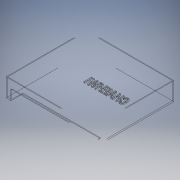
# Autodesk Inventor part: 240621_뚜껑
Saved by Autodesk Inventor 2016 (Build 200138000, 138)
## iProperties
Created: 2024-06-21
Part Number: 240621_뚜껑
Material: 일반
Document SubType Name: Modeling
Designer: pc
Density: 1 g/cm^3
Appearance: 기본값
Author: pc
Autodesk Inventor part; units mm, degrees
ref_plane "YZ Plane" through (0, 0, 0) normal (1, 0, 0) x (0, 1, 0)
ref_plane "XZ Plane" through (0, 0, 0) normal (0, 1, 0) x (-1, 0, 0)
ref_plane "XY Plane" through (0, 0, 0) normal (0, 0, 1) x (1, 0, 0)
sketch "스케치1" plane through (0, 0, 0) normal (0, 0, 1) x (1, 0, 0)
  line L0 (67, -62) -> (-67, -62)
  line L1 (-67, -62) -> (-67, 62)
  line L2 (-67, 62) -> (67, 62)
  line L3 (67, 62) -> (67, -62)
  line L4 (67, -62) -> (-67, 62) construction
  line L5 (-67, -62) -> (67, 62) construction
  point P0 (0, 0)
  dimension "d0" = 134
  dimension "d1" = 124
  constraints: 12 end point, 2 midpoint, 2 parallel, 1 horizontal, 1 perpendicular
  measures "d0" distance of L1.end L2.end
  measures "d1" distance of L0.end L1.end
extrude "돌출1" add sketch "스케치1" along normal blind 28
shell "쉘1" thickness 1.2 removed faces 1 at (22.3333, 20.6667, 28)
sketch "스케치2" plane through (0, 0, 0) normal (0, 0, -1) x (-1, 0, 0)
  line L0 (59.4523, -61.8902) -> (-59.4523, -61.8902)
  line L1 (-59.4523, -61.8902) -> (-59.4523, -43.79)
  line L2 (-59.4523, -43.79) -> (59.4523, -43.79)
  line L3 (59.4523, -43.79) -> (59.4523, -61.8902)
  line L4 (59.4523, -61.8902) -> (-59.4523, -43.79) construction
  line L5 (-59.4523, -61.8902) -> (59.4523, -43.79) construction
  point P0 (0, 0)
  point P1 (0, -52.8401)
  constraints: 12 end point, 2 midpoint, 2 parallel, 1 horizontal, 1 perpendicular
extrude "돌출2" cut sketch "스케치2" against normal blind 1.2
sketch "스케치3" plane through (0, 0, 0) normal (0, 0, -1) x (-1, 0, 0)
  line L0 (-31.3452, 31.9819) -> (-10.2317, 31.9819) construction
  line L1 (-10.2317, 31.9819) -> (-10.2317, 28.3571) construction
  line L2 (-10.2317, 28.3571) -> (-31.3452, 28.3571) construction
  line L3 (-31.3452, 28.3571) -> (-31.3452, 31.9819) construction
  spline S0 degree 2 poles (-23.1755, 23.6344) (-23.1755, 23.7476) (-23.1755, 23.9819) (-23.2078, 24.1597) knots 0 0 0 1 2 2 2
  line L4 (-23.2078, 24.1597) -> (-24.7432, 24.1597)
  spline S1 degree 2 poles (-24.7432, 24.1597) (-24.7432, 23.1981) (-25.325, 20.7657) (-26.7714, 20.7657) knots 0 0 0 1 2 2 2
  spline S2 degree 2 poles (-26.7714, 20.7657) (-28.3068, 20.8789) (-28.9129, 23.8122) (-28.9129, 25.4284) knots 0 0 0 1 2 2 2
  spline S3 degree 2 poles (-28.9129, 25.4284) (-28.9129, 25.5496) (-28.9129, 25.7758) (-28.9129, 25.8971) knots 0 0 0 1 2 2 2
  spline S4 degree 2 poles (-28.9129, 25.8971) (-28.9129, 27.0849) (-28.3472, 30.5597) (-26.828, 30.5597) knots 0 0 0 1 2 2 2
  spline S5 degree 2 poles (-26.828, 30.5597) (-25.4219, 30.5597) (-24.7432, 28.79) (-24.7432, 27.8364) knots 0 0 0 1 2 2 2
  line L5 (-24.7432, 27.8364) -> (-23.2078, 27.8364)
  spline S6 degree 2 poles (-23.2078, 27.8364) (-23.1755, 27.9819) (-23.1755, 28.1516) (-23.1755, 28.2162) knots 0 0 0 1 2 2 2
  spline S7 degree 2 poles (-23.1755, 28.2162) (-23.1755, 30.4142) (-25.325, 31.9819) (-26.6098, 31.9819) knots 0 0 0 1 2 2 2
  spline S8 degree 2 poles (-26.6098, 31.9819) (-29.4785, 31.893) (-30.4805, 27.4001) (-30.4805, 25.4284) knots 0 0 0 1 2 2 2
  spline S9 degree 2 poles (-30.4805, 25.4284) (-30.4805, 22.8829) (-29.131, 19.4567) (-26.6098, 19.3435) knots 0 0 0 1 2 2 2
  spline S10 degree 2 poles (-26.6098, 19.3435) (-24.7512, 19.3435) (-23.1755, 21.9536) (-23.1755, 23.6344) knots 0 0 0 1 2 2 2
  line L6 (-14.0765, 19.6021) -> (-14.0765, 31.6021)
  line L7 (-14.0765, 31.6021) -> (-15.6442, 31.6021)
  line L8 (-15.6442, 31.6021) -> (-15.6442, 26.7617)
  line L9 (-15.6442, 26.7617) -> (-19.927, 26.7617)
  line L10 (-19.927, 26.7617) -> (-19.927, 31.6021)
  line L11 (-19.927, 31.6021) -> (-21.4947, 31.6021)
  line L12 (-21.4947, 31.6021) -> (-21.4947, 19.6021)
  line L13 (-21.4947, 19.6021) -> (-19.927, 19.6021)
  line L14 (-19.927, 19.6021) -> (-19.927, 25.3395)
  line L15 (-19.927, 25.3395) -> (-15.6442, 25.3395)
  line L16 (-15.6442, 25.3395) -> (-15.6442, 19.6021)
  line L17 (-15.6442, 19.6021) -> (-14.0765, 19.6021)
  line L18 (-4.1371, 19.6021) -> (-7.4098, 31.6021)
  line L19 (-7.4098, 31.6021) -> (-9.4381, 31.6021)
  line L20 (-9.4381, 31.6021) -> (-12.7997, 19.6021)
  line L21 (-12.7997, 19.6021) -> (-11.1512, 19.6021)
  line L22 (-11.1512, 19.6021) -> (-10.2785, 22.9637)
  line L23 (-10.2785, 22.9637) -> (-6.6826, 22.9637)
  line L24 (-6.6826, 22.9637) -> (-5.8421, 19.6021)
  line L25 (-5.8421, 19.6021) -> (-4.1371, 19.6021)
  line L26 (-7.1189, 24.3859) -> (-9.8421, 24.3859)
  line L27 (-9.8421, 24.3859) -> (-8.4846, 30.0102)
  line L28 (-8.4846, 30.0102) -> (-7.1189, 24.3859)
  line L29 (3.4023, 30.1799) -> (3.4023, 31.6021)
  line L30 (3.4023, 31.6021) -> (-2.8603, 31.6021)
  line L31 (-2.8603, 31.6021) -> (-2.8603, 19.6021)
  line L32 (-2.8603, 19.6021) -> (3.2892, 19.6021)
  line L33 (3.2892, 19.6021) -> (3.2892, 21.0243)
  line L34 (3.2892, 21.0243) -> (-1.2927, 21.0243)
  line L35 (-1.2927, 21.0243) -> (-1.2927, 25.2263)
  line L36 (-1.2927, 25.2263) -> (3.0548, 25.2263)
  line L37 (3.0548, 25.2263) -> (3.0548, 26.6486)
  line L38 (3.0548, 26.6486) -> (-1.2927, 26.6486)
  line L39 (-1.2927, 26.6486) -> (-1.2927, 30.1799)
  line L40 (-1.2927, 30.1799) -> (3.4023, 30.1799)
  line L41 (12.2346, 19.6021) -> (12.2346, 31.6021)
  line L42 (12.2346, 31.6021) -> (10.6669, 31.6021)
  line L43 (10.6669, 31.6021) -> (10.6669, 26.7617)
  line L44 (10.6669, 26.7617) -> (6.3841, 26.7617)
  line L45 (6.3841, 26.7617) -> (6.3841, 31.6021)
  line L46 (6.3841, 31.6021) -> (4.8164, 31.6021)
  line L47 (4.8164, 31.6021) -> (4.8164, 19.6021)
  line L48 (4.8164, 19.6021) -> (6.3841, 19.6021)
  line L49 (6.3841, 19.6021) -> (6.3841, 25.3395)
  line L50 (6.3841, 25.3395) -> (10.6669, 25.3395)
  line L51 (10.6669, 25.3395) -> (10.6669, 19.6021)
  line L52 (10.6669, 19.6021) -> (12.2346, 19.6021)
  line L53 (26.1174, 31.6021) -> (24.5821, 31.6021)
  line L54 (24.5821, 31.6021) -> (22.6427, 21.7193)
  line L55 (22.6427, 21.7193) -> (20.7518, 31.6021)
  line L56 (20.7518, 31.6021) -> (19.0144, 31.6021)
  line L57 (19.0144, 31.6021) -> (16.9619, 21.7758)
  line L58 (16.9619, 21.7758) -> (15.1599, 31.6021)
  line L59 (15.1599, 31.6021) -> (13.5114, 31.6021)
  line L60 (13.5114, 31.6021) -> (16.0003, 19.6021)
  line L61 (16.0003, 19.6021) -> (17.8831, 19.6021)
  line L62 (17.8831, 19.6021) -> (19.8306, 29.687)
  line L63 (19.8306, 29.687) -> (21.7134, 19.6021)
  line L64 (21.7134, 19.6021) -> (23.5962, 19.6021)
  line L65 (23.5962, 19.6021) -> (26.1174, 31.6021)
  line L66 (29.1882, 19.6021) -> (29.1882, 31.6021)
  line L67 (29.1882, 31.6021) -> (27.6205, 31.6021)
  line L68 (27.6205, 31.6021) -> (27.6205, 19.6021)
  line L69 (27.6205, 19.6021) -> (29.1882, 19.6021)
  point P0 (0, 0)
  dimension "d0" = 134
  dimension "d1" = 124
  constraints: 2 other
extrude "돌출3" add sketch "스케치3" along normal blind 2
sketch "스케치5" plane through (-67, -62, 0) normal (0, -1, 0) x (1, 0, 0)
  line L0 (7.5477, 0) -> (126.4523, 0) projected
  line L1 (126.4523, 0) -> (7.5477, 0)
  line L2 (7.5477, 0) -> (7.5477, 15.3269)
  line L3 (7.5477, 15.3269) -> (126.4523, 15.3269)
  line L4 (126.4523, 15.3269) -> (126.4523, 0)
  point P0 (67, 0)
  constraints: 8 end point, 2 parallel, 1 horizontal, 1 perpendicular
extrude "돌출5" cut sketch "스케치5" against normal blind 1.2
sketch "스케치6" plane through (67, -62, 0) normal (1, 0, 0) x (0, 0, -1)
  line L0 (-28, 0) -> (-28, 124) construction
  line L1 (-28, 124) -> (-25, 124) construction
  line L2 (0, 124) -> (-28, 124) construction
  line L3 (-25, 124) -> (-25, 114) construction
  circle A0 centre (-25, 114) radius 1.75
  line L4 (-28, 0) -> (-25, 0) construction
  line L5 (0, 0) -> (-28, 0) construction
  line L6 (-25, 0) -> (-25, 10) construction
  circle A1 centre (-25, 10) radius 1.75
  point P0 (0, 62)
  dimension "d13" = 3
  dimension "d14" = 10
  dimension "d15" = 3.5
  dimension "d16" = 3
  dimension "d17" = 10
  dimension "d18" = 3.5
  constraints: 8 end point, 2 centre point, 2 coincident, 2 point on line, 1 vertical
  measures "d13" distance of L0.end L1.end
  measures "d14" distance of L1.end L3.end
  measures "d15" diameter of A0
  measures "d16" distance of L0.start L4.end
  measures "d17" distance of L4.end L6.end
  measures "d18" diameter of A1
extrude "돌출6" cut sketch "스케치6" against normal blind 200
